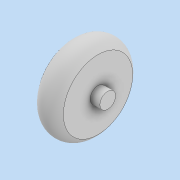
# Autodesk Inventor part: wheel
Saved by Autodesk Inventor 2022 (Build 260153000, 153)
## iProperties
Created: 2022-09-24
Part Number: wheel
Material: Générique
Document SubType Name: Modeling
Designer: andre
Density: 1 g/cm^3
Appearance: Par défaut
Author: andre
Autodesk Inventor part; units mm, degrees
ref_plane "YZ Plane" through (0, 0, 0) normal (1, 0, 0) x (0, 1, 0)
ref_plane "XZ Plane" through (0, 0, 0) normal (0, 1, 0) x (-1, 0, 0)
ref_plane "XY Plane" through (0, 0, 0) normal (0, 0, 1) x (1, 0, 0)
sketch "Esquisse1" plane through (0, 0, 0) normal (0, 1, 0) x (-1, 0, 0)
  line L0 (0, 0) -> (0, 4.75)
  line L1 (0, 4.75) -> (5.9, 4.75)
  line L2 (5.9, 4.75) -> (5.9, 21)
  arc A0 (21.5, 21) -> (5.9, 21) centre (13.7, 16.2864) ccw
  line L3 (21.5, 21) -> (21.5, 0)
  line L4 (21.5, 0) -> (0, 0)
  line L5 (13.7, 25.4) -> (29.3742, 25.4)
  line L6 (0, 0) -> (27.0366, 0)
  dimension "d0" = 4.75
  dimension "d1" = 5.9
  dimension "d2" = 15.6
  dimension "d3" = 25.4
  dimension "d4" = 21
  constraints: 14 end point, 3 perpendicular, 3 point on circle, 2 vertical, 1 centre point, 1 horizontal, 1 point on line, 1 tangent
  measures "d0" distance between parallel lines of L4 L1
  measures "d1" distance of L0.end L1.end
  measures "d2" distance between parallel lines of L2 L3
  measures "d3" distance between parallel lines of L5 L6
  measures "d4" distance of L3.start L3.end
revolve "Révolution1" add sketch "Esquisse1" angle 360 about axis through (0, 0, 0) along (-1, 0, 0)
